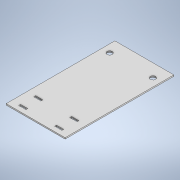
# Autodesk Inventor part: Platte1
Saved by Autodesk Inventor 2022 (Build 260153000, 153)
## iProperties
Created: 2022-04-02
Part Number: Platte1
Material: Generic
Document SubType Name: Modeling
Designer: benni
Density: 1 g/cm^3
Appearance: Default
Author: benni
Autodesk Inventor part; units mm, degrees
ref_plane "YZ Plane" through (0, 0, 0) normal (1, 0, 0) x (0, 1, 0)
ref_plane "XZ Plane" through (0, 0, 0) normal (0, 1, 0) x (-1, 0, 0)
ref_plane "XY Plane" through (0, 0, 0) normal (0, 0, 1) x (1, 0, 0)
sketch "Sketch1" plane through (0, 0, 0) normal (0, 1, 0) x (-1, 0, 0)
  line L0 (0, 0) -> (45, 0)
  line L1 (45, 0) -> (45, -83)
  line L2 (45, -83) -> (0, -83)
  line L3 (0, -83) -> (0, 0)
  circle A0 centre (39, -73) radius 2
  line L4 (22.5, 0) -> (22.5, -83)
  circle A1 centre (6, -73) radius 2
  line L5 (45, -10) -> (0, -10)
  line L6 (6, -3.5) -> (11.525, -3.5)
  line L7 (11.525, -3.5) -> (11.525, -5)
  line L8 (11.525, -5) -> (6, -5)
  line L9 (6, -5) -> (6, -3.5)
  line L10 (6, -16.5) -> (11.525, -16.5)
  line L11 (11.525, -16.5) -> (11.525, -15)
  line L12 (11.525, -15) -> (6, -15)
  line L13 (6, -15) -> (6, -16.5)
  line L14 (39, -3.5) -> (33.475, -3.5)
  line L15 (33.475, -3.5) -> (33.475, -5)
  line L16 (33.475, -5) -> (39, -5)
  line L17 (39, -5) -> (39, -3.5)
  line L18 (39, -16.5) -> (33.475, -16.5)
  line L19 (33.475, -15) -> (39, -15)
  line L20 (39, -15) -> (39, -16.5)
  line L21 (33.475, -16.5) -> (33.475, -15)
  dimension "d0" = 45
  dimension "d1" = 83
  dimension "d2" = 10
  dimension "d3" = 6
  dimension "d9" = 4
  dimension "d13" = 45
  dimension "d22" = 20
  dimension "d23" = 6
  dimension "d24" = 10
  dimension "d25" = 1.5
  constraints: 44 end point, 13 symmetric about line, 4 parallel, 4 perpendicular, 2 centre point, 2 horizontal, 2 midpoint, 2 point on line, 1 coincident, 1 other
  measures "d0" distance of L1.end L2.end
  measures "d1" distance of L0.end L1.end
  measures "d2" distance from line of L2 point (39, -73)
  measures "d3" distance from line of L1 point (39, -73)
  measures "d9" diameter of A0
  measures "d13" diameter of L3 L4
  measures "d22" diameter of L0 L5
  measures "d23" distance between parallel lines of L3 L9
  measures "d24" diameter of L8 L5
  measures "d25" distance of L6.end L7.end
extrude "Extrusion3" add sketch "Sketch1" along normal blind 1
equation "\"d13\" = d0"
body "Solid3"
